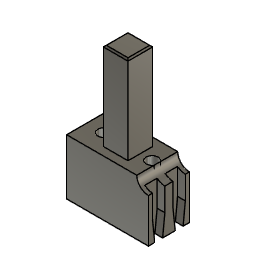
Wheel truing stand (copy) (Autodesk Fusion 360 archive; units mm, degrees)
design "Non_movable_piece"
Autodesk Fusion 360 part; units mm, degrees
(part 1 of 2)
sketch "Sketch1" plane through (0, 0, 0) normal (0, 1, 0) x (1, 0, 0)
  line L0 (0, 0) -> (56, 0)
  line L1 (56, 0) -> (56, -38)
  line L2 (56, -38) -> (0, -38)
  line L3 (0, -38) -> (0, 0)
  line L4 (56, 0) -> (56, -1.6379)
  line L5 (56, 0) -> (56, -30)
  circle A0 centre (56, -38) radius 8
  dimension "d1" = 56
  dimension "d2" = 38
  dimension "d5" = 30
  constraint horizontal L0
  constraint vertical L1
  constraint horizontal L2
  constraint vertical L3
  constraint coincident L0.start L3.end
  constraint coincident L1 L4.end
  constraint perpendicular L0 L5
  constraint coincident L1.end L2.start
  constraint coincident L5.end A0
  measures "d1" distance of L0.start L0.end
  measures "d2" distance of L0.start L2.end
  measures "d5" distance of L0.end L5.end
  measures "d8" distance of L0.start
  measures "d9" distance of L0.start
extrude "Extrude1" add sketch "Sketch1" along normal blind 28 contours L0 L1 L2 L3 L4 L5 A0
sketch "Sketch3" plane through (0, 0, 38) normal (0, 0, 1) x (-1, 0, 0)
  line L0 (0, 0) -> (-48, 0)
  line L1 (-48, 0) -> (-48, -28)
  line L2 (-48, -28) -> (0, -28)
  line L3 (0, -28) -> (0, 0)
  line L4 (0, -28) -> (-56, -28)
  line L5 (-56, -28) -> (-56, 0)
  line L6 (-56, 0) -> (0, 0)
  line L7 (0, 0) -> (0, -28)
  line L8 (-56, -28) -> (0, 0) construction
  line L9 (0, -28) -> (-56, 0) construction
  line L10 (-36.4, -5.6) -> (-19.6, -5.6)
  line L11 (-19.6, -5.6) -> (-19.6, -22.4)
  line L12 (-19.6, -22.4) -> (-36.4, -22.4)
  line L13 (-36.4, -22.4) -> (-36.4, -5.6)
  line L14 (-36.4, -5.6) -> (-19.6, -22.4) construction
  line L15 (-19.6, -5.6) -> (-36.4, -22.4) construction
  line L16 (0, -14) -> (-56, -14) construction
  line L17 (0, -14) -> (-11.5, -14)
  line L18 (-56, -14) -> (-44.5, -14)
  circle A0 centre (-11.5, -14) radius 2
  line L19 (-28, 0) -> (-28, -28) construction
  circle A1 centre (-44.5, -14) radius 2
  circle A2 centre (-11.5, -14) radius 4.1
  circle A3 centre (-44.5, -14) radius 4.1
  line L20 (-38.15, -3.85) -> (-17.85, -3.85)
  line L21 (-17.85, -3.85) -> (-17.85, -24.15)
  line L22 (-17.85, -24.15) -> (-38.15, -24.15)
  line L23 (-38.15, -24.15) -> (-38.15, -3.85)
  line L24 (-38.15, -3.85) -> (-17.85, -24.15) construction
  line L25 (-17.85, -3.85) -> (-38.15, -24.15) construction
  line L26 (-16.35, -2.35) -> (-16.35, -25.65)
  line L27 (-16.35, -25.65) -> (-39.65, -25.65)
  line L28 (-39.65, -25.65) -> (-39.65, -2.35)
  line L29 (-39.65, -2.35) -> (-16.35, -2.35)
  point P0 (-28, -14)
  point P1 (-28, -14)
  dimension "d6" = 56
  dimension "d7" = 28
  dimension "d8" = 16.8
  dimension "d9" = 16.8
  dimension "d13" = 11.5
  dimension "d14" = 11.5
  dimension "d15" = 4
  dimension "d17" = 8.2
  dimension "d33" = 20.3
  dimension "d34" = 20.3
  dimension "d35" = -1.5
  constraint horizontal L4
  constraint vertical L5
  constraint horizontal L6
  constraint vertical L7
  constraint coincident L2.end L3.start
  constraint coincident L0.start L3.end
  constraint horizontal L10
  constraint perpendicular L10 L11
  constraint parallel L10 L12
  constraint parallel L11 L13
  constraint coincident L14 P1
  constraint coincident L15 P1
  constraint midpoint L8 P1
  constraint midpoint L7 L16.start
  constraint midpoint L5 L16.end
  constraint perpendicular L11 L17
  constraint perpendicular L1 L18
  constraint coincident L17.end A0.centre
  constraint midpoint L6 L19.start
  constraint midpoint L4 L19.end
  constraint symmetric A0 L19 A1
  constraint symmetric L19 A2 A3
  constraint horizontal L20
  constraint perpendicular L20 L21
  constraint parallel L20 L22
  constraint parallel L21 L23
  constraint coincident L24 P1
  constraint coincident L25 P1
  constraint coincident P1 P0
  measures "d6" distance of L5 L7
  measures "d7" distance of L4 L6
  measures "d8" distance of L11.end L12.end
  measures "d9" distance of L10.end L11.end
  measures "d13" distance of L16.start L17.end
  measures "d14" distance of L16.end L18.end
  measures "d15" diameter of A0
  measures "d17" diameter of A2
  measures "d33" distance of L21.end L22.end
  measures "d34" distance of L20.end L21.end
extrude "Extrude3" cut sketch "Sketch3" against normal blind 38 contours A0 | A1
extrude "Extrude2" add sketch "Sketch3" along normal blind 60 contours L10 L11 L12 L13
chamfer "Chamfer1" distance 1 angle 45 4 edges at (28, 5.6, 98) (19.6, 14, 98) (28, 22.4, 98) (36.4, 14, 98)
extrude "Extrude4" cut sketch "Sketch3" against normal blind 32 contours L1 A3 | A2
chamfer "Chamfer2" distance 1.8 angle 45 2 edges at (13.3647, 14.7232, 6) (46.3647, 14.7232, 6)
sketch "Sketch4" plane through (56, 0, 0) normal (1, 0, 0) x (0, 1, 0)
  line L0 (0, 30) -> (0, 0)
  line L1 (0, 0) -> (28, 0)
  line L2 (28, 0) -> (28, 30)
  line L3 (28, 30) -> (0, 30)
  line L4 (0, 38) -> (28, 38) construction
  line L5 (28, 38) -> (28, 0) construction
  line L6 (28, 0) -> (0, 0) construction
  line L7 (0, 0) -> (0, 38) construction
  line L8 (14, 0) -> (14, 38) construction
  line L9 (7, 0) -> (7, 38) construction
  line L10 (7, 0) -> (4.5, 0)
  line L11 (7, 14) -> (3, 14)
  line L12 (3, 14) -> (4.5, 0)
  line L13 (7, 14) -> (11, 14)
  line L14 (11, 14) -> (9.5, 0)
  line L15 (7, 0) -> (9.5, 0)
  line L16 (7, 14.2) -> (2.7774, 14.2)
  line L17 (2.7774, 14.2) -> (4.3203, -0.2)
  line L18 (7, -0.2) -> (4.3203, -0.2)
  line L19 (7, -0.2) -> (9.6797, -0.2)
  line L20 (11.2226, 14.2) -> (9.6797, -0.2)
  line L21 (7, 14.2) -> (11.2226, 14.2)
  line L22 (2.7774, 14.2) -> (2.7774, 38)
  line L23 (11.2226, 14.2) -> (11.2226, 38.0127)
  line L24 (16.7774, 14.2) -> (16.7774, 38.0127)
  line L25 (25.2226, 14.2) -> (25.2226, 38)
  line L26 (16.7774, 14.2) -> (18.3203, -0.2)
  line L27 (25.2226, 14.2) -> (23.6797, -0.2)
  line L28 (21, -0.2) -> (23.6797, -0.2)
  line L29 (21, -0.2) -> (18.3203, -0.2)
  line L30 (16.7774, 38.0127) -> (25.2226, 38)
  line L31 (11.2226, 38.0127) -> (2.7774, 38)
  dimension "d24" = 2.5
  dimension "d25" = 4
  dimension "d27" = 14
  dimension "d28" = 0.2
  dimension "d29" = 180
  dimension "d30" = 23.8127
  constraint horizontal L4
  constraint vertical L5
  constraint horizontal L6
  constraint vertical L7
  constraint coincident L1.end L2.start
  constraint midpoint L1 L8.start
  constraint midpoint L4 L8.end
  constraint perpendicular L4 L8
  constraint coincident L1 L9.start
  constraint coincident L4 L9.end
  constraint perpendicular L4 L9
  constraint perpendicular L9 L10
  constraint coincident L9 L11.start
  constraint perpendicular L9 L11
  constraint symmetric L10.start L9 L15.start
  constraint symmetric L9 L10.end L14.end
  constraint symmetric L9 L11.start L13.start
  constraint symmetric L9 L11.end L13.end
  constraint vertical L22
  constraint coincident L4 L22.end
  constraint symmetric L8 L16.end L25.start
  constraint symmetric L8 L17.end L27.end
  constraint symmetric L8 L18.start L28.start
  constraint symmetric L8 L19.end L26.end
  constraint symmetric L8 L20.start L24.start
  constraint symmetric L8 L22.end L25.end
  constraint symmetric L8 L23.end L24.end
  measures "d24" distance of L9.start L10.end
  measures "d25" distance of L11.start L11.end
  measures "d27" distance of L10 L11
  measures "d29" angle of L22 L23
  measures "d30" distance of L20.start L23.end
extrude "Extrude5" cut sketch "Sketch4" against normal blind 5.3 contours L3 L22 L23 L31 | L3 L16 L21 L22 L23 | L1 L11 L12 L13 L14 L16 L17 L20 L21 | L1 L10 L11 L12 L13 L14 L15 | L3 L24 L25 L30 | L1 L3 L24 L25 L26 L27
equation "d13 = ( 23 / 2 ) * 1 mm"
equation "d14 = ( 23 / 2 ) * 1 mm"

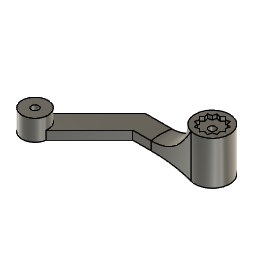
design "wheel_aligment_arm_right_20mm_offset"
Autodesk Fusion 360 part; units mm, degrees
sketch "Sketch1" plane through (0, 0, 0) normal (0, 0, 1) x (1, 0, 0)
  line L0 (0, 0) -> (40, 0)
  line L1 (40, 12) -> (0, 12)
  line L2 (0, 12) -> (0, 0)
  line L3 (40, 0) -> (68.2843, -28.2843)
  line L4 (40, 0) -> (80, 0) construction
  line L5 (68.2843, -28.2843) -> (76.7696, -19.799)
  line L6 (76.7696, -19.799) -> (44.9706, 12)
  line L7 (40, 12) -> (44.9706, 12)
  circle A0 centre (0, 6) radius 10
  line L8 (0, 6) -> (0, 13.5) construction
  line L9 (0, 13.5) -> (0, -1.5) construction
  line L10 (0, 6) -> (7.5, 6) construction
  line L11 (7.5, 6) -> (-7.5, 6) construction
  line L12 (-7.5, 6) -> (0, 13.5)
  line L13 (0, 13.5) -> (7.5, 6)
  line L14 (7.5, 6) -> (0, -1.5)
  line L15 (0, -1.5) -> (-7.5, 6)
  line L16 (0, 6) -> (3.75, 12.4952) construction
  line L17 (3.75, 12.4952) -> (-3.75, -0.4952) construction
  line L18 (0, 6) -> (6.4952, 2.25) construction
  line L19 (6.4952, 2.25) -> (-6.4952, 9.75) construction
  line L20 (-6.4952, 9.75) -> (3.75, 12.4952)
  line L21 (3.75, 12.4952) -> (6.4952, 2.25)
  line L22 (6.4952, 2.25) -> (-3.75, -0.4952)
  line L23 (-3.75, -0.4952) -> (-6.4952, 9.75)
  line L24 (0, 6) -> (6.4952, 9.75) construction
  line L25 (0, 6) -> (7.5, 6) construction
  line L26 (6.4952, 9.75) -> (-6.4952, 2.25) construction
  line L27 (0, 6) -> (3.75, -0.4952) construction
  line L28 (3.75, -0.4952) -> (-3.75, 12.4952) construction
  line L29 (-3.75, 12.4952) -> (-6.4952, 2.25)
  line L30 (-6.4952, 2.25) -> (3.75, -0.4952)
  line L31 (3.75, -0.4952) -> (6.4952, 9.75)
  line L32 (6.4952, 9.75) -> (-3.75, 12.4952)
  circle A1 centre (0, 6) radius 2
  circle A2 centre (72.5269, -24.0416) radius 7.5
  line L33 (76.1769, -26.149) -> (76.1769, -21.9343)
  line L34 (76.1769, -21.9343) -> (72.5269, -19.827)
  line L35 (72.5269, -19.827) -> (68.8769, -21.9343)
  line L36 (68.8769, -21.9343) -> (68.8769, -26.149)
  line L37 (68.8769, -26.149) -> (72.5269, -28.2563)
  line L38 (72.5269, -28.2563) -> (76.1769, -26.149)
  line L39 (68.8769, -21.9343) -> (68.8769, -17.4897)
  line L40 (76.1769, -21.9343) -> (76.1769, -17.4897)
  circle A3 centre (72.5269, -24.0416) radius 2.1
  point P0 (72.5269, -24.0416)
  dimension "d1" = 40
  dimension "d2" = 12
  dimension "d3" = 40
  dimension "d4" = 45
  dimension "d5" = 12
  dimension "d8" = 7.5
  dimension "d9" = 15
  dimension "d10" = 7.5
  dimension "d11" = 15
  dimension "d12" = 7.5
  dimension "d13" = 30
  dimension "d14" = 15
  dimension "d15" = 7.5
  dimension "d16" = 90
  dimension "d17" = 15
  dimension "d18" = 30
  dimension "d19" = 7.5
  dimension "d20" = 15
  dimension "d21" = 7.5
  dimension "d22" = 15
  dimension "d23" = 20
  dimension "d24" = 4
  dimension "d25" = 15
  dimension "d35" = 3.65
  dimension "d39" = 4.2
  dimension "d42" = 180
  constraint horizontal L0
  constraint horizontal L1
  constraint vertical L2
  constraint coincident L0.start L2.end
  constraint horizontal L4
  constraint perpendicular L3 L5
  constraint perpendicular L5 L6
  constraint midpoint L2 A0.centre
  constraint coincident A0.centre L8.start
  constraint parallel L2 L8
  constraint perpendicular L0 L9
  constraint perpendicular L8 L10
  constraint parallel L10 L11
  constraint parallel L16 L17
  constraint perpendicular L16 L19
  constraint horizontal L25
  constraint parallel L24 L26
  constraint perpendicular L24 L27
  constraint parallel L27 L28
  constraint midpoint L5 P0
  constraint coincident P0 A2.centre
  constraint vertical L39
  constraint coincident A2 L39.end
  constraint vertical L40
  constraint coincident A2 L40.end
  measures "d1" distance of L0.start L0.end
  measures "d2" distance of L0.start L1.end
  measures "d3" distance of L0.end L3.end
  measures "d4" angle of L3 L4
  measures "d5" distance of L3.end L5.end
  measures "d8" distance of A0.centre L8.end
  measures "d9" distance of L8.end L9.end
  measures "d10" distance of A0.centre L10.end
  measures "d11" distance of L10.end L11.end
  measures "d12" distance of A0.centre L16.end
  measures "d13" angle of L9 L16
  measures "d14" distance of L16.end L17.end
  measures "d15" distance of A0.centre L18.end
  measures "d16" angle of L17 L18
  measures "d17" distance of L18.end L19.end
  measures "d18" angle of L24 L25
  measures "d19" distance of A0.centre L24.end
  measures "d20" distance of L24.end L26.end
  measures "d21" distance of A0.centre L27.end
  measures "d22" distance of L27.end L28.end
  measures "d23" diameter of A0
  measures "d24" diameter of A1
  measures "d25" diameter of A2
  measures "d35" distance of P0 L38
  measures "d39" diameter of A3
  measures "d42" angle of L36 L39 L0.start
extrude "Extrude1" add sketch "Sketch1" against normal blind 5
extrude "Extrude9" add sketch "Sketch1" against normal blind 25 contours L0 L2 L14 L30 | L0 L2 L14 L15 L22 | L0 L14 L30 | L0 L1 A0 L12 L13 L14 L15 L20 L21 L22 L23 L29 L30 L31 L32 | L2 L12 L15 L20 L23 L29 L30 A1 | L2 L13 L14 L21 L22 L31 L32 A1 | L15 L22 L30 | L14 L22 L30 | L0 L14 L22 L30 L31 | L0 L30 L31 | L2 A1 | L2 A1 | L14 L22 L31 | L15 L22 L23 L30 | L15 L23 L30 | L0 L1 A0 L13 L14 L21 L22 L31 L32 | L14 L21 L31 | L14 L21 L22 L31 | L15 L23 L29 L30 | L15 L23 L29 | L1 L2 L12 L13 L32 | L1 L2 L13 L20 | L13 L20 L32 | L12 L20 L32 | L13 L14 L21 L31 | L13 L21 L31 | L12 L15 L23 L29 | L12 L23 L29 | L12 L20 L29 L32 | L12 L20 L29 | L1 L13 L20 L21 L32 | L1 L13 L20 | L13 L21 L32 | L13 L21 L31 L32 | L12 L20 L23 L29 | L1 L20 L21
extrude "Extrude2" cut sketch "Sketch1" along normal blind 2.2 from surface at -25 contours L0 L2 L14 L30 | L0 L2 L14 L15 L22 | L0 L14 L30 | L2 L12 L15 L20 L23 L29 L30 A1 | L2 L13 L14 L21 L22 L31 L32 A1 | L15 L22 L30 | L14 L22 L30 | L0 L14 L22 L30 L31 | L0 L30 L31 | L2 A1 | L2 A1 | L14 L22 L31 | L15 L22 L23 L30 | L15 L23 L30 | L14 L21 L31 | L14 L21 L22 L31 | L15 L23 L29 L30 | L15 L23 L29 | L1 L2 L12 L13 L32 | L1 L2 L13 L20 | L13 L20 L32 | L12 L20 L32 | L13 L14 L21 L31 | L13 L21 L31 | L12 L15 L23 L29 | L12 L23 L29 | L12 L20 L29 L32 | L12 L20 L29 | L1 L13 L20 L21 L32 | L1 L13 L20 | L13 L21 L32 | L13 L21 L31 L32 | L12 L20 L23 L29 | L1 L20 L21
extrude "Extrude3" cut sketch "Sketch1" against normal blind 25 contours L2 A1 | L2 A1
extrude "Extrude4" add sketch "Sketch1" against normal blind 12 contours L3 L5 A2 L36 L37 L39 | L3 L5 L6 A2 L33 L37 L38 L40 | L5 L6 A2 L34 L35 L39 L40 | L5 L34 L35 L36 L37 A3 | L5 L33 L34 L37 L38 A3 | L6 A2 L40 | L5 A3 | L5 A3 | L5 L6 L40 | L5 L34 L40
extrude "Extrude5" cut sketch "Sketch1" along normal mid plane 4 from surface at -7 contours L5 L6 A2 L34 L35 L39 L40 | L5 L34 L35 L36 L37 A3 | L5 L33 L34 L37 L38 A3 | L6 A2 L40 | L5 A3 | L5 A3 | L5 L34 L40
extrude "Extrude6" cut sketch "Sketch1" against normal blind 12 contours L5 A3 | L5 A3
move_body "Move1" bodies 1 to x (-1, 0, 0) y (0, 1, 0) z (0, 0, -1) at (-20, 0, -50)
move_body "Move2" bodies 1 to x (1, 0, 0) y (0, 1, 0) z (0, 0, 1) at (20, 0, 50)
move_body "Move3" bodies 1 to x (1, 0, 0) y (0, 1, 0) z (0, 0, 1) at (-0.21, 0.1034, 0.1851)
fillet "Fillet1" radius 20 1 edges at (-10.21, 6.1034, 5.1851)
fillet "Fillet2" radius 100 2 edges at (-8.21, 0.1034, 12.6851) (-8.21, 12.1034, 12.6851)
equation "d13 = ( 90 / 3 ) * 1 deg"

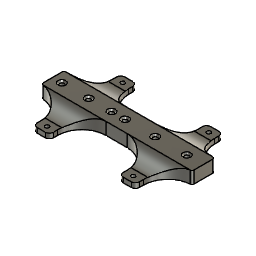
design "base"
Autodesk Fusion 360 part; units mm, degrees
sketch "Sketch1" plane through (0, 0, 0) normal (0, 0, 1) x (1, 0, 0)
  line L0 (0, 0) -> (186, 0)
  line L1 (186, 0) -> (186, 28)
  line L2 (186, 28) -> (0, 28)
  line L3 (0, 28) -> (0, 0)
  line L4 (0, 14) -> (186, 14) construction
  circle A0 centre (11.5, 14) radius 2.75
  circle A1 centre (44.5, 14) radius 2.75
  circle A2 centre (72.6667, 14) radius 2.75
  circle A3 centre (89.3333, 14) radius 2.75
  circle A4 centre (126.5, 14) radius 2.75
  circle A5 centre (165.5, 14) radius 2.75
  line L5 (13.8094, 10) -> (16.1188, 14)
  line L6 (16.1188, 14) -> (13.8094, 18)
  line L7 (13.8094, 18) -> (9.1906, 18)
  line L8 (9.1906, 18) -> (6.8812, 14)
  line L9 (6.8812, 14) -> (9.1906, 10)
  line L10 (9.1906, 10) -> (13.8094, 10)
  line L11 (46.8094, 10) -> (49.1188, 14)
  line L12 (49.1188, 14) -> (46.8094, 18)
  line L13 (46.8094, 18) -> (42.1906, 18)
  line L14 (42.1906, 18) -> (39.8812, 14)
  line L15 (39.8812, 14) -> (42.1906, 10)
  line L16 (42.1906, 10) -> (46.8094, 10)
  line L17 (74.9761, 10) -> (77.2855, 14)
  line L18 (77.2855, 14) -> (74.9761, 18)
  line L19 (74.9761, 18) -> (70.3573, 18)
  line L20 (70.3573, 18) -> (68.0479, 14)
  line L21 (68.0479, 14) -> (70.3573, 10)
  line L22 (70.3573, 10) -> (74.9761, 10)
  line L23 (91.6427, 10) -> (93.9521, 14)
  line L24 (93.9521, 14) -> (91.6427, 18)
  line L25 (91.6427, 18) -> (87.0239, 18)
  line L26 (87.0239, 18) -> (84.7145, 14)
  line L27 (84.7145, 14) -> (87.0239, 10)
  line L28 (87.0239, 10) -> (91.6427, 10)
  line L29 (128.8094, 10) -> (131.1188, 14)
  line L30 (131.1188, 14) -> (128.8094, 18)
  line L31 (128.8094, 18) -> (124.1906, 18)
  line L32 (124.1906, 18) -> (121.8812, 14)
  line L33 (121.8812, 14) -> (124.1906, 10)
  line L34 (124.1906, 10) -> (128.8094, 10)
  line L35 (167.8094, 10) -> (170.1188, 14)
  line L36 (170.1188, 14) -> (167.8094, 18)
  line L37 (167.8094, 18) -> (163.1906, 18)
  line L38 (163.1906, 18) -> (160.8812, 14)
  line L39 (160.8812, 14) -> (163.1906, 10)
  line L40 (163.1906, 10) -> (167.8094, 10)
  point P0 (11.5, 14)
  point P1 (44.5, 14)
  point P2 (72.6667, 14)
  point P3 (89.3333, 14)
  point P4 (126.5, 14)
  point P5 (165.5, 14)
  dimension "d1" = 186
  dimension "d2" = 28
  dimension "d3" = 5.5
  dimension "d4" = 11.5
  dimension "d5" = 5.5
  dimension "d6" = 44.5
  dimension "d7" = 5.5
  dimension "d8" = 5.5
  dimension "d9" = 5.5
  dimension "d10" = 5.5
  dimension "d11" = 72.6667
  dimension "d12" = 89.3333
  dimension "d13" = 20.5
  dimension "d14" = 126.5
  dimension "d18" = 4
  dimension "d19" = 4
  dimension "d20" = 4
  dimension "d21" = 4
  dimension "d22" = 4
  dimension "d23" = 4
  constraint horizontal L0
  constraint vertical L1
  constraint horizontal L2
  constraint vertical L3
  constraint coincident L0.start L3.end
  constraint midpoint L3 L4.start
  constraint midpoint L1 L4.end
  constraint coincident L4 P0
  constraint coincident L4 P1
  constraint coincident L4 P2
  constraint coincident L4 P3
  constraint coincident L4 P4
  constraint coincident L4 P5
  constraint coincident P0 A0.centre
  constraint coincident P1 A1.centre
  constraint coincident P2 A2.centre
  constraint coincident P3 A3.centre
  constraint coincident P4 A4.centre
  constraint coincident P5 A5.centre
  measures "d1" distance of L0.start L0.end
  measures "d2" distance of L0.start L2.end
  measures "d3" diameter of A0
  measures "d4" distance of L4.start P0
  measures "d5" diameter of A1
  measures "d6" distance of L3 P1
  measures "d7" diameter of A2
  measures "d8" diameter of A3
  measures "d9" diameter of A4
  measures "d10" diameter of A5
  measures "d11" distance of L3 P2
  measures "d12" distance of L3 P3 L0.start
  measures "d13" distance of L1 P5
  measures "d14" distance of L3 P4
  measures "d18" distance of P0 L10
  measures "d19" distance of P1 L16
  measures "d20" distance of P2 L22
  measures "d21" distance of P3 L28
  measures "d22" distance of P4 L34
  measures "d23" distance of P5 L40
extrude "Extrude1" add sketch "Sketch1" along normal blind 15 contours L0 L1 L2 L3 | L5 L6 L7 L8 L9 L10 | L11 L12 L13 L14 L15 L16 | L17 L18 L19 L20 L21 L22 | L23 L24 L25 L26 L27 L28 | L29 L30 L31 L32 L33 L34 | L35 L36 L37 L38 L39 L40
chamfer "Chamfer1" distance 2 angle 45 6 edges at (8.9361, 14.9944, 15) (41.9361, 14.9944, 15) (70.1028, 14.9944, 15) (86.7694, 14.9944, 15) (123.9361, 14.9944, 15) (162.9361, 14.9944, 15)
extrude "Extrude2" cut sketch "Sketch1" along normal blind 4 contours L5 L6 L7 L8 L9 L10 | L11 L12 L13 L14 L15 L16 | L17 L18 L19 L20 L21 L22 | L23 L24 L25 L26 L27 L28 | L29 L30 L31 L32 L33 L34 | L35 L36 L37 L38 L39 L40
sketch "Sketch2" plane through (0, 0, 0) normal (-1, 0, 0) x (0, -1, 0)
  line L0 (-28, 0) -> (0, 0)
  line L1 (0, 0) -> (0, 15)
  line L2 (0, 15) -> (-28, 15)
  line L3 (-28, 15) -> (-28, 0)
  line L4 (0, 0) -> (40, 0)
  line L5 (40, 0) -> (40, 6)
  line L6 (40, 6) -> (25, 6)
  arc A0 (0, 15) -> (25, 6) centre (25, 45.2222) ccw
  line L7 (0, 15) -> (-28, 0) construction
  line L8 (-28, 15) -> (0, 0) construction
  line L9 (-14, -17.2562) -> (-14, 34) construction
  line L10 (-28, 0) -> (-68, 0)
  arc A1 (-53, 6) -> (-28, 15) centre (-53, 45.2222) ccw
  line L11 (-68, 6) -> (-53, 6)
  line L12 (-68, 0) -> (-68, 6)
  dimension "d26" = 40
  constraint coincident L0.end L1.start
  constraint perpendicular L1 L4
  constraint perpendicular L4 L5
  constraint perpendicular L5 L6
  constraint tangent L6 A0
  constraint coincident L1.end L2.start
  constraint coincident L0.start L3.end
  constraint coincident L2.end L3.start
  constraint perpendicular L2 L9
  constraint symmetric L0.end L9 L0.start
  constraint symmetric L4.end L9 L10.end
  constraint symmetric L5.end L9 L11.start
  constraint symmetric L6.end L9 A1.start
  constraint symmetric L1.end L9 L2.end
  constraint symmetric A0 L9 A1
  measures "d26" distance of L0.end L4.end
extrude "Extrude3" add sketch "Sketch2" against normal blind 20 from surface at -30 contours L3 L10 A1 L11 L12 | L1 L4 L5 L6 A0
extrude "Extrude4" add sketch "Sketch2" along normal blind 20 from surface at -156 contours L3 L10 A1 L11 L12 | L1 L4 L5 L6 A0
fillet "Fillet1" radius 30 8 edges at (50, 0, 7.5) (30, 0, 7.5) (50, 28, 7.5) (136, 28, 7.5) (156, 28, 7.5) (156, 0, 7.5) (136, 0, 7.5) (30, 28, 7.5)
sketch "Sketch3" plane through (0, 0, 6) normal (0, 0, 1) x (-1, 0, 0)
  line L0 (-30, 30) -> (-30, 40)
  line L1 (-30, 40) -> (-50, 40)
  line L2 (-50, 40) -> (-50, 30)
  arc A0 (-50.4196, 25) -> (-50, 30) centre (-80, 30) ccw
  line L3 (-50.4196, 25) -> (-29.5804, 25)
  arc A1 (-30, 30) -> (-29.5804, 25) centre (0, 30) ccw
  line L4 (-156, 40) -> (-156, 30)
  arc A2 (-156.4196, 25) -> (-156, 30) centre (-186, 30) ccw
  line L5 (-156.4196, 25) -> (-135.5804, 25)
  arc A3 (-136, 30) -> (-135.5804, 25) centre (-106, 30) ccw
  line L6 (-136, 30) -> (-136, 40)
  line L7 (-136, 40) -> (-156, 40)
  line L8 (-156, -58) -> (-156, -68)
  line L9 (-156, -68) -> (-136, -68)
  line L10 (-136, -68) -> (-136, -58)
  arc A4 (-135.5804, -53) -> (-136, -58) centre (-106, -58) ccw
  line L11 (-135.5804, -53) -> (-156.4196, -53)
  arc A5 (-156, -58) -> (-156.4196, -53) centre (-186, -58) ccw
  line L12 (-30, -68) -> (-30, -58)
  arc A6 (-29.5804, -53) -> (-30, -58) centre (0, -58) ccw
  line L13 (-29.5804, -53) -> (-50.4196, -53)
  arc A7 (-50, -58) -> (-50.4196, -53) centre (-80, -58) ccw
  line L14 (-50, -58) -> (-50, -68)
  line L15 (-50, -68) -> (-30, -68)
  line L16 (-50.4196, 25) -> (-30, 40) construction
  line L17 (-29.5804, 25) -> (-50, 40) construction
  line L18 (-156, -68) -> (-135.5804, -53) construction
  line L19 (-136, -68) -> (-156.4196, -53) construction
  line L20 (-136, 40) -> (-156.4196, 25) construction
  line L21 (-135.5804, 25) -> (-156, 40) construction
  line L22 (-29.5804, -53) -> (-50, -68) construction
  line L23 (-30, -68) -> (-50.4196, -53) construction
  circle A8 centre (-40, -60.6541) radius 2.5
  circle A9 centre (-40, 32.6541) radius 2.5
  circle A10 centre (-146, 32.6541) radius 2.5
  circle A11 centre (-146, -60.6541) radius 2.5
  point P0 (-146, 32.6541)
  point P1 (-146, -60.6541)
  dimension "d35" = 5
  dimension "d36" = 5
  dimension "d37" = 5
  dimension "d38" = 5
  constraint coincident A0.start L3.start
  constraint coincident L0.end L1.start
  constraint coincident L3.end A1.end
  constraint coincident L1.end L2.start
  constraint coincident L8.end L9.start
  constraint coincident A4.start L11.start
  constraint coincident L9.end L10.start
  constraint coincident L11.end A5.end
  constraint coincident L6.end L7.start
  constraint coincident A2.start L5.start
  constraint coincident L5.end A3.end
  constraint coincident L4.start L7.end
  constraint coincident L21 P0
  constraint coincident L20 P0
  constraint coincident L18 P1
  constraint coincident L19 P1
  constraint coincident A6.start L13.start
  constraint coincident L14.end L15.start
  constraint coincident L12.start L15.end
  constraint coincident L13.end A7.end
  constraint coincident L22 A8.centre
  constraint coincident L23 A8.centre
  constraint coincident L17 A9.centre
  constraint coincident L16 A9.centre
  constraint coincident P0 A10.centre
  constraint coincident P1 A11.centre
  measures "d35" diameter of A8
  measures "d36" diameter of A9
  measures "d37" diameter of A10
  measures "d38" diameter of A11
extrude "Extrude5" cut sketch "Sketch3" against normal blind 6 contours A8 | A9 | A10 | A11
fillet "Fillet2" radius 2.5 4 edges at (186, 0, 7.5) (186, 28, 7.5) (0, 0, 7.5) (0, 28, 7.5)
fillet "Fillet3" radius 5 8 edges at (30, -40, 3) (50, -40, 3) (136, -40, 3) (156, -40, 3) (156, 68, 3) (136, 68, 3) (50, 68, 3) (30, 68, 3)
equation "d1 = 50 mm + 56 mm + 80 mm"
equation "d11 = 56 mm + ( 50 / 3 ) * 1 mm"
equation "d12 = 56 mm + ( 2 * 50 / 3 ) * 1 mm"
equation "d14 = 106 mm + 20.5 mm"
equation "d30 = -186 mm + 30.00 mm"

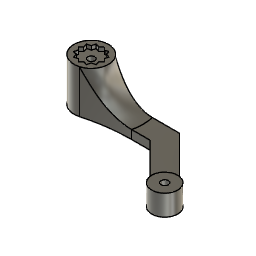
design "wheel_aligment_arm_left_20mm_offset"
Autodesk Fusion 360 part; units mm, degrees
sketch "Sketch1" plane through (0, 0, 0) normal (0, 0, 1) x (1, 0, 0)
  line L0 (0, 0) -> (40, 0)
  line L1 (40, 12) -> (0, 12)
  line L2 (0, 12) -> (0, 0)
  line L3 (40, 0) -> (68.2843, -28.2843)
  line L4 (40, 0) -> (80, 0) construction
  line L5 (68.2843, -28.2843) -> (76.7696, -19.799)
  line L6 (76.7696, -19.799) -> (44.9706, 12)
  line L7 (40, 12) -> (44.9706, 12)
  circle A0 centre (0, 6) radius 10
  line L8 (0, 6) -> (0, 13.5) construction
  line L9 (0, 13.5) -> (0, -1.5) construction
  line L10 (0, 6) -> (7.5, 6) construction
  line L11 (7.5, 6) -> (-7.5, 6) construction
  line L12 (-7.5, 6) -> (0, 13.5)
  line L13 (0, 13.5) -> (7.5, 6)
  line L14 (7.5, 6) -> (0, -1.5)
  line L15 (0, -1.5) -> (-7.5, 6)
  line L16 (0, 6) -> (3.75, 12.4952) construction
  line L17 (3.75, 12.4952) -> (-3.75, -0.4952) construction
  line L18 (0, 6) -> (6.4952, 2.25) construction
  line L19 (6.4952, 2.25) -> (-6.4952, 9.75) construction
  line L20 (-6.4952, 9.75) -> (3.75, 12.4952)
  line L21 (3.75, 12.4952) -> (6.4952, 2.25)
  line L22 (6.4952, 2.25) -> (-3.75, -0.4952)
  line L23 (-3.75, -0.4952) -> (-6.4952, 9.75)
  line L24 (0, 6) -> (6.4952, 9.75) construction
  line L25 (0, 6) -> (7.5, 6) construction
  line L26 (6.4952, 9.75) -> (-6.4952, 2.25) construction
  line L27 (0, 6) -> (3.75, -0.4952) construction
  line L28 (3.75, -0.4952) -> (-3.75, 12.4952) construction
  line L29 (-3.75, 12.4952) -> (-6.4952, 2.25)
  line L30 (-6.4952, 2.25) -> (3.75, -0.4952)
  line L31 (3.75, -0.4952) -> (6.4952, 9.75)
  line L32 (6.4952, 9.75) -> (-3.75, 12.4952)
  circle A1 centre (0, 6) radius 2
  circle A2 centre (72.5269, -24.0416) radius 7.5
  line L33 (76.1769, -26.149) -> (76.1769, -21.9343)
  line L34 (76.1769, -21.9343) -> (72.5269, -19.827)
  line L35 (72.5269, -19.827) -> (68.8769, -21.9343)
  line L36 (68.8769, -21.9343) -> (68.8769, -26.149)
  line L37 (68.8769, -26.149) -> (72.5269, -28.2563)
  line L38 (72.5269, -28.2563) -> (76.1769, -26.149)
  line L39 (68.8769, -21.9343) -> (68.8769, -17.4897)
  line L40 (76.1769, -21.9343) -> (76.1769, -17.4897)
  circle A3 centre (72.5269, -24.0416) radius 2.1
  point P0 (72.5269, -24.0416)
  dimension "d1" = 40
  dimension "d2" = 12
  dimension "d3" = 40
  dimension "d4" = 45
  dimension "d5" = 12
  dimension "d8" = 7.5
  dimension "d9" = 15
  dimension "d10" = 7.5
  dimension "d11" = 15
  dimension "d12" = 7.5
  dimension "d13" = 30
  dimension "d14" = 15
  dimension "d15" = 7.5
  dimension "d16" = 90
  dimension "d17" = 15
  dimension "d18" = 30
  dimension "d19" = 7.5
  dimension "d20" = 15
  dimension "d21" = 7.5
  dimension "d22" = 15
  dimension "d23" = 20
  dimension "d24" = 4
  dimension "d25" = 15
  dimension "d35" = 3.65
  dimension "d39" = 4.2
  dimension "d42" = 180
  constraint horizontal L0
  constraint horizontal L1
  constraint vertical L2
  constraint coincident L0.start L2.end
  constraint horizontal L4
  constraint perpendicular L3 L5
  constraint perpendicular L5 L6
  constraint midpoint L2 A0.centre
  constraint coincident A0.centre L8.start
  constraint parallel L2 L8
  constraint perpendicular L0 L9
  constraint perpendicular L8 L10
  constraint parallel L10 L11
  constraint parallel L16 L17
  constraint perpendicular L16 L19
  constraint horizontal L25
  constraint parallel L24 L26
  constraint perpendicular L24 L27
  constraint parallel L27 L28
  constraint midpoint L5 P0
  constraint coincident P0 A2.centre
  constraint vertical L39
  constraint coincident A2 L39.end
  constraint vertical L40
  constraint coincident A2 L40.end
  measures "d1" distance of L0.start L0.end
  measures "d2" distance of L0.start L1.end
  measures "d3" distance of L0.end L3.end
  measures "d4" angle of L3 L4
  measures "d5" distance of L3.end L5.end
  measures "d8" distance of A0.centre L8.end
  measures "d9" distance of L8.end L9.end
  measures "d10" distance of A0.centre L10.end
  measures "d11" distance of L10.end L11.end
  measures "d12" distance of A0.centre L16.end
  measures "d13" angle of L9 L16
  measures "d14" distance of L16.end L17.end
  measures "d15" distance of A0.centre L18.end
  measures "d16" angle of L17 L18
  measures "d17" distance of L18.end L19.end
  measures "d18" angle of L24 L25
  measures "d19" distance of A0.centre L24.end
  measures "d20" distance of L24.end L26.end
  measures "d21" distance of A0.centre L27.end
  measures "d22" distance of L27.end L28.end
  measures "d23" diameter of A0
  measures "d24" diameter of A1
  measures "d25" diameter of A2
  measures "d35" distance of P0 L38
  measures "d39" diameter of A3
  measures "d42" angle of L36 L39 L0.start
extrude "Extrude1" add sketch "Sketch1" along normal blind 5
extrude "Extrude7" add sketch "Sketch1" along normal blind 25 contours L0 L2 L14 L30 | L0 L2 L14 L15 L22 | L0 L14 L30 | L0 L1 A0 L12 L13 L14 L15 L20 L21 L22 L23 L29 L30 L31 L32 | L2 L12 L15 L20 L23 L29 L30 A1 | L2 L13 L14 L21 L22 L31 L32 A1 | L15 L22 L30 | L14 L22 L30 | L0 L14 L22 L30 L31 | L0 L30 L31 | L2 A1 | L2 A1 | L14 L22 L31 | L15 L22 L23 L30 | L15 L23 L30 | L0 L1 A0 L13 L14 L21 L22 L31 L32 | L14 L21 L31 | L14 L21 L22 L31 | L15 L23 L29 L30 | L15 L23 L29 | L1 L2 L12 L13 L32 | L1 L2 L13 L20 | L13 L20 L32 | L12 L20 L32 | L13 L14 L21 L31 | L13 L21 L31 | L12 L15 L23 L29 | L12 L23 L29 | L12 L20 L29 L32 | L12 L20 L29 | L1 L13 L20 L21 L32 | L1 L13 L20 | L13 L21 L32 | L13 L21 L31 L32 | L12 L20 L23 L29 | L1 L20 L21
extrude "Extrude2" cut sketch "Sketch1" against normal blind 2.2 from surface at 25 contours L0 L2 L14 L30 | L0 L2 L14 L15 L22 | L0 L14 L30 | L2 L12 L15 L20 L23 L29 L30 A1 | L2 L13 L14 L21 L22 L31 L32 A1 | L15 L22 L30 | L14 L22 L30 | L0 L14 L22 L30 L31 | L0 L30 L31 | L2 A1 | L2 A1 | L14 L22 L31 | L15 L22 L23 L30 | L15 L23 L30 | L14 L21 L31 | L14 L21 L22 L31 | L15 L23 L29 L30 | L15 L23 L29 | L1 L2 L12 L13 L32 | L1 L2 L13 L20 | L13 L20 L32 | L12 L20 L32 | L13 L14 L21 L31 | L13 L21 L31 | L12 L15 L23 L29 | L12 L23 L29 | L12 L20 L29 L32 | L12 L20 L29 | L1 L13 L20 L21 L32 | L1 L13 L20 | L13 L21 L32 | L13 L21 L31 L32 | L12 L20 L23 L29 | L1 L20 L21
extrude "Extrude3" cut sketch "Sketch1" along normal blind 22.8 contours L2 A1 | L2 A1
extrude "Extrude4" add sketch "Sketch1" along normal blind 12 contours L3 L5 A2 L36 L37 L39 | L3 L5 L6 A2 L33 L37 L38 L40 | L5 L6 A2 L34 L35 L39 L40 | L5 L34 L35 L36 L37 A3 | L5 L33 L34 L37 L38 A3 | L6 A2 L40 | L5 A3 | L5 A3 | L5 L6 L40 | L5 L34 L40
extrude "Extrude5" cut sketch "Sketch1" along normal mid plane 4 from surface at 7 contours L5 L6 A2 L34 L35 L39 L40 | L5 L34 L35 L36 L37 A3 | L5 L33 L34 L37 L38 A3 | L6 A2 L40 | L5 A3 | L5 A3 | L5 L34 L40
extrude "Extrude6" cut sketch "Sketch1" along normal blind 14 contours L5 A3 | L5 A3
fillet "Fillet1" radius 20 1 edges at (10, 6, 5)
fillet "Fillet2" radius 100 2 edges at (8, 0, 12.5) (8, 12, 12.5)
equation "d13 = ( 90 / 3 ) * 1 deg"

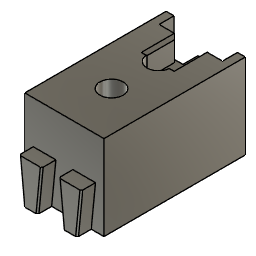
design "Connector_piece"
Autodesk Fusion 360 part; units mm, degrees
sketch "Sketch1" plane through (0, 0, 0) normal (0, 1, 0) x (1, 0, 0)
  line L0 (0, 0) -> (28, 0)
  line L1 (28, 0) -> (28, -30)
  line L2 (28, -30) -> (0, -30)
  line L3 (0, -30) -> (0, 0)
  dimension "d1" = 28
  dimension "d2" = 30
  constraint horizontal L0
  constraint vertical L1
  constraint horizontal L2
  constraint vertical L3
  constraint coincident L0.start L3.end
  measures "d1" distance of L0.start L0.end
  measures "d2" distance of L0.start L2.end
extrude "Extrude1" add sketch "Sketch1" along normal blind 50
sketch "Sketch3" plane through (0, 0, 30) normal (0, 0, 1) x (-1, 0, 0)
  line L0 (0, 0) -> (-28, 0)
  line L1 (-28, 0) -> (-28, -50)
  line L2 (-28, -50) -> (0, -50)
  line L3 (0, -50) -> (0, 0)
  line L4 (0, -16.6667) -> (-28, -16.6667)
  line L5 (0, -33.3333) -> (-28, -33.3333)
  circle A0 centre (-14, -33.3333) radius 2
  circle A1 centre (-14, -16.6667) radius 2
  circle A2 centre (-14, -16.6667) radius 4.1
  circle A3 centre (-14, -33.3333) radius 4.1
  dimension "d25" = 16.6667
  dimension "d26" = 16.6667
  dimension "d27" = 4
  dimension "d28" = 4
  dimension "d29" = 8.2
  dimension "d30" = 8.2
  constraint coincident L3 L4.start
  constraint coincident L1 L4.end
  constraint perpendicular L1 L4
  constraint coincident L3 L5.start
  constraint coincident L1 L5.end
  constraint perpendicular L1 L5
  constraint midpoint L5 A0.centre
  constraint midpoint L4 A1.centre
  constraint concentric A1 A2
  constraint concentric A0 A3
  measures "d25" distance of L0 L4
  measures "d26" distance of L2 L5
  measures "d27" diameter of A0
  measures "d28" diameter of A1
  measures "d29" diameter of A2
  measures "d30" diameter of A3
extrude "Extrude5" cut sketch "Sketch3" against normal blind 30 contours L4 A1 | L4 A1 | L5 A0 | L5 A0
sketch "Sketch2" plane through (0, 50, 0) normal (0, 1, 0) x (-1, 0, 0)
  line L0 (0, 30) -> (-28, 30)
  line L1 (-28, 30) -> (-28, 0)
  line L2 (-28, 0) -> (0, 0)
  line L3 (0, 0) -> (0, 30)
  line L4 (-28, 30) -> (-14, 30) construction
  line L5 (-14, 30) -> (-14, 0) construction
  line L6 (-14, 0) -> (-28, 0) construction
  line L7 (-28, 0) -> (-28, 30) construction
  line L8 (-21, 30) -> (-21, 0) construction
  line L9 (-21, 0) -> (-23.5, 0)
  line L10 (-21, 0) -> (-18.5, 0)
  line L11 (-21, 15) -> (-25, 15)
  line L12 (-25, 15) -> (-23.5, 0)
  line L13 (-21, 0) -> (-18.5, 0)
  line L14 (-21, 0) -> (-23.5, 0)
  line L15 (-17, 15) -> (-18.5, 0)
  line L16 (-21, 15) -> (-17, 15)
  line L17 (-11, 15) -> (-9.5, 0)
  line L18 (-7, 15) -> (-11, 15)
  line L19 (-7, 15) -> (-3, 15)
  line L20 (-3, 15) -> (-4.5, 0)
  line L21 (-7, 0) -> (-4.5, 0)
  line L22 (-7, 0) -> (-9.5, 0)
  line L23 (-21, 15.5) -> (-16.4475, 15.5)
  line L24 (-16.4475, 15.5) -> (-18.0475, -0.5)
  line L25 (-21, -0.5) -> (-18.0475, -0.5)
  line L26 (-21, -0.5) -> (-23.9525, -0.5)
  line L27 (-25.5525, 15.5) -> (-23.9525, -0.5)
  line L28 (-21, 15.5) -> (-25.5525, 15.5)
  line L29 (-7, -0.5) -> (-9.9525, -0.5)
  line L30 (-11.5525, 15.5) -> (-9.9525, -0.5)
  line L31 (-7, 15.5) -> (-11.5525, 15.5)
  line L32 (-7, 15.5) -> (-2.4475, 15.5)
  line L33 (-2.4475, 15.5) -> (-4.0475, -0.5)
  line L34 (-7, -0.5) -> (-4.0475, -0.5)
  line L35 (-25.5525, 15.5) -> (-25.5525, 30)
  line L36 (-2.4475, 15.5) -> (-2.4475, 30)
  line L37 (-16.4475, 15.5) -> (-16.4475, 30)
  line L38 (-11.5525, 15.5) -> (-11.5525, 30)
  line L39 (-28, 30) -> (-28, 22)
  line L40 (0, 30) -> (0, 22)
  line L41 (0, 22) -> (-9.2, 22)
  line L42 (-28, 22) -> (-18.8, 22)
  line L43 (-18.8, 22) -> (-18.8, 30)
  line L44 (-9.2, 22) -> (-9.2, 30)
  line L45 (-18.8, 22) -> (-9.2, 22)
  line L46 (-7, 15.2) -> (-11.221, 15.2)
  line L47 (-11.221, 15.2) -> (-9.681, -0.2)
  line L48 (-7, -0.2) -> (-9.681, -0.2)
  line L49 (-7, -0.2) -> (-4.319, -0.2)
  line L50 (-2.779, 15.2) -> (-4.319, -0.2)
  line L51 (-7, 15.2) -> (-2.779, 15.2)
  line L52 (-21, 15.2) -> (-16.779, 15.2)
  line L53 (-16.779, 15.2) -> (-18.319, -0.2)
  line L54 (-21, -0.2) -> (-18.319, -0.2)
  line L55 (-21, -0.2) -> (-23.681, -0.2)
  line L56 (-25.221, 15.2) -> (-23.681, -0.2)
  line L57 (-21, 15.2) -> (-25.221, 15.2)
  line L58 (-25.221, 15.2) -> (-25.221, 30)
  line L59 (-16.779, 15.2) -> (-16.779, 30)
  line L60 (-11.221, 15.2) -> (-11.221, 30)
  line L61 (-2.779, 15.2) -> (-2.779, 30)
  dimension "d5" = 2.5
  dimension "d6" = 2.5
  dimension "d7" = 4
  dimension "d8" = 15
  dimension "d9" = -0.5
  dimension "d16" = 8
  dimension "d17" = 8
  dimension "d18" = 9.2
  dimension "d19" = 9.2
  dimension "d20" = 8
  dimension "d37" = 0.2
  dimension "d38" = 0.2
  dimension "d39" = 180
  constraint horizontal L4
  constraint vertical L5
  constraint horizontal L6
  constraint vertical L7
  constraint midpoint L2 L5.end
  constraint coincident L0.end L1.start
  constraint midpoint L4 L8.start
  constraint midpoint L6 L8.end
  constraint perpendicular L8 L9
  constraint perpendicular L8 L10
  constraint coincident L8 L11.start
  constraint perpendicular L8 L11
  constraint symmetric L9.start L8 L10.start
  constraint symmetric L8 L9.end L10.end
  constraint symmetric L8 L10.end L9.end
  constraint symmetric L8 L11.start L16.start
  constraint symmetric L8 L11.end L15.start
  constraint symmetric L5 L8.end L21.start
  constraint symmetric L5 L9.end L20.end
  constraint symmetric L5 L11.start L18.start
  constraint symmetric L5 L11.end L19.end
  constraint symmetric L5 L10.end L17.end
  constraint symmetric L5 L15.start L17.start
  constraint vertical L35
  constraint coincident L4 L35.end
  constraint symmetric L5 L27.start L32.end
  constraint symmetric L5 L35.end L36.end
  constraint symmetric L8 L27.start L23.end
  constraint symmetric L8 L35.end L37.end
  constraint symmetric L5 L23.end L30.start
  constraint symmetric L5 L37.end L38.end
  constraint perpendicular L4 L39
  constraint coincident L0.start L3.end
  constraint perpendicular L0 L40
  constraint perpendicular L40 L41
  constraint perpendicular L35 L42
  constraint vertical L43
  constraint coincident L0 L44.end
  constraint perpendicular L0 L44
  constraint vertical L58
  constraint coincident L4 L58.end
  constraint coincident L4 L59.end
  constraint symmetric L5 L52.end L46.end
  constraint symmetric L5 L56.start L50.start
  constraint symmetric L5 L58.end L61.end
  constraint symmetric L5 L59.end L60.end
  measures "d5" distance of L8.end L9.end
  measures "d6" distance of L8.end L10.end
  measures "d7" distance of L11.start L11.end
  measures "d8" distance of L9 L11
  measures "d16" distance of L0.end L39.end
  measures "d17" distance of L0.start L40.end
  measures "d18" distance of L40.end L41.end
  measures "d19" distance of L39.end L42.end
  measures "d20" distance of L42.end L43.end
  measures "d39" angle of L58 L59
extrude "Extrude6" cut sketch "Sketch3" against normal blind 24 contours L4 A1 A2 | L4 A1 A2 | L5 A0 A3 | L5 A0 A3
chamfer "Chamfer4" distance 1.8 angle 45 2 edges at (15.8647, 34.0566, 6) (15.8647, 17.3899, 6)
extrude "Extrude4" cut sketch "Sketch2" against normal blind 16 contours L0 L44 L45 L60 | L0 L38 L45 L60 | L0 L37 L38 L45 | L0 L37 L45 L59 | L0 L43 L45 L59
extrude "Extrude3" add sketch "Sketch2" against normal blind 5 from surface at -50 contours L2 L17 L18 L19 L20 L21 L22 | L2 L9 L10 L11 L12 L13 L14 L15 L16
chamfer "Chamfer1" distance 0.5 angle 45 4 edges at (3.75, -5, 7.5) (10.25, -5, 7.5) (17.75, -5, 7.5) (24.25, -5, 7.5)
extrude "Extrude2" cut sketch "Sketch2" against normal blind 5.3 contours L0 L41 L44 L61 | L0 L44 L45 L60 | L31 L32 L41 L45 L60 L61 | L31 L32 L46 L51 L60 L61 | L2 L17 L18 L19 L20 L46 L47 L50 L51 | L2 L17 L18 L19 L20 L21 L22 | L0 L43 L45 L59 | L0 L42 L43 L58 | L23 L28 L42 L45 L58 L59 | L23 L28 L52 L57 L58 L59 | L2 L9 L10 L13 L14 L53 L54 L55 L56 | L2 L11 L12 L15 L16 L52 L53 L56 L57 | L2 L9 L10 L11 L12 L13 L14 L15 L16
chamfer "Chamfer2" distance 1 angle 45 4 edges at (18.8, 39.35, 30) (18.4227, 34, 30) (9.5773, 34, 30) (9.2, 39.35, 30)
chamfer "Chamfer3" distance 1 angle 45 2 edges at (18.8, 44.7, 25.5) (9.2, 44.7, 25.5)
chamfer "Chamfer6" distance 0.7 angle 45 2 edges at (18.0454, 34, 25.5) (9.9546, 34, 25.5)
ref_plane "WorkPlane1" through (14, 25, 15) normal (1, 0, 0) x (0, 0, -1)
equation "d25 = ( 50 / 3 ) * 1 mm"
equation "d26 = ( 50 / 3 ) * 1 mm"

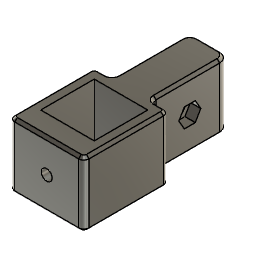
design "Pin_height_adjuster"
Autodesk Fusion 360 part; units mm, degrees
sketch "Sketch1" plane through (0, 0, 0) normal (0, 0, 1) x (1, 0, 0)
  line L0 (10, -10) -> (-10, -10)
  line L1 (-10, -10) -> (-10, 10)
  line L2 (-10, 10) -> (10, 10)
  line L3 (10, 10) -> (10, -10)
  line L4 (10, -10) -> (-10, 10) construction
  line L5 (-10, -10) -> (10, 10) construction
  line L6 (10.3, -10.3) -> (-10.3, -10.3)
  line L7 (-10.3, -10.3) -> (-10.3, 10.3)
  line L8 (-10.3, 10.3) -> (10.3, 10.3)
  line L9 (10.3, 10.3) -> (10.3, -10.3)
  line L10 (-14.3, -14.3) -> (-14.3, 14.3)
  line L11 (-14.3, 14.3) -> (14.3, 14.3)
  line L12 (14.3, 14.3) -> (14.3, -14.3)
  line L13 (14.3, -14.3) -> (-14.3, -14.3)
  line L14 (-14.3, -14.3) -> (14.3, -14.3)
  line L15 (14.3, -14.3) -> (14.3, -18.3)
  line L16 (14.3, -18.3) -> (-14.3, -18.3)
  line L17 (-14.3, -18.3) -> (-14.3, -14.3)
  dimension "d1" = 20
  dimension "d2" = 20
  dimension "d3" = -0.3
  dimension "d4" = -4.3
  dimension "d10" = 28.6
  dimension "d11" = 4
  constraint horizontal L0
  constraint perpendicular L0 L1
  constraint parallel L0 L2
  constraint parallel L1 L3
  constraint coincident L4 origin
  constraint coincident L5 origin
  constraint horizontal L14
  constraint vertical L15
  constraint horizontal L16
  constraint vertical L17
  measures "d1" distance of L1.end L2.end
  measures "d2" distance of L0.end L1.end
  measures "d10" distance of L10.start L12.end
  measures "d11" distance of L10.start L16.end
extrude "Extrude1" add sketch "Sketch1" along normal blind 25 contours L10 L11 L12 L13 L14 | L13 L14 L15 L16 L17
sketch "Sketch3" plane through (0, -10.3, 0) normal (0, 1, 0) x (-1, 0, 0)
  line L0 (-10.3, 0) -> (10.3, 0)
  line L1 (10.3, 0) -> (10.3, 25)
  line L2 (10.3, 25) -> (-10.3, 25)
  line L3 (-10.3, 25) -> (-10.3, 0)
  line L4 (-10.3, 25) -> (10.3, 25)
  line L5 (10.3, 25) -> (10.3, 0)
  line L6 (10.3, 0) -> (-10.3, 0)
  line L7 (-10.3, 0) -> (-10.3, 25)
  line L8 (-10.3, 25) -> (10.3, 0) construction
  line L9 (10.3, 25) -> (-10.3, 0) construction
  line L10 (2.1073, 8.85) -> (4.2147, 12.5)
  line L11 (4.2147, 12.5) -> (2.1073, 16.15)
  line L12 (2.1073, 16.15) -> (-2.1073, 16.15)
  line L13 (-2.1073, 16.15) -> (-4.2147, 12.5)
  line L14 (-4.2147, 12.5) -> (-2.1073, 8.85)
  line L15 (-2.1073, 8.85) -> (2.1073, 8.85)
  circle A0 centre (0, 12.5) radius 2.1
  point P0 (0, 12.5)
  dimension "d12" = 25
  dimension "d13" = 3.65
  dimension "d16" = 4.2
  constraint horizontal L4
  constraint vertical L5
  constraint horizontal L6
  constraint vertical L7
  constraint coincident L2.end L3.start
  constraint coincident L0.end L1.start
  constraint midpoint L9 P0
  constraint coincident P0 A0.centre
  measures "d12" distance of L2.end L0.start
  measures "d13" distance of P0 L15
  measures "d16" diameter of A0
extrude "Extrude4" cut sketch "Sketch3" against normal blind 8 contours A0
extrude "Extrude3" cut sketch "Sketch3" against normal blind 4 contours L10 L11 L12 L13 L14 L15 | A0
sketch "Sketch6" plane through (0, 14.3, 0) normal (0, 1, 0) x (-1, 0, 0)
  line L0 (-14.3, 0) -> (14.3, 0)
  line L1 (14.3, 0) -> (14.3, 25)
  line L2 (14.3, 25) -> (-14.3, 25)
  line L3 (-14.3, 25) -> (-14.3, 0)
  line L4 (-14.3, 25) -> (14.3, 0) construction
  line L5 (14.3, 25) -> (-14.3, 0) construction
  line L6 (7.5, 25) -> (-7.5, 25)
  line L7 (-7.5, 25) -> (-7.5, 0)
  line L8 (-7.5, 0) -> (7.5, 0)
  line L9 (7.5, 0) -> (7.5, 25)
  line L10 (7.5, 25) -> (-7.5, 0) construction
  line L11 (-7.5, 25) -> (7.5, 0) construction
  point P0 (0, 12.5)
  dimension "d35" = 15
  dimension "d36" = 25
  constraint coincident L2.end L3.start
  constraint coincident L0.end L1.start
  constraint coincident L1.end L2.start
  constraint coincident L0.start L3.end
  constraint horizontal L6
  constraint perpendicular L6 L7
  constraint parallel L6 L8
  constraint parallel L7 L9
  constraint coincident L10 P0
  constraint coincident L11 P0
  constraint midpoint L5 P0
  measures "d35" distance of L7.end L8.end
  measures "d36" distance of L6.end L7.end
extrude "Extrude10" add sketch "Sketch6" along normal blind 30 contours L0 L2 L6 L7 L8 L9
sketch "Sketch7" plane through (-7.5, 0, 0) normal (-1, 0, 0) x (0, -1, 0)
  line L0 (-14.3, 0) -> (-14.3, 25)
  line L1 (-14.3, 25) -> (-44.3, 25)
  line L2 (-44.3, 25) -> (-44.3, 0)
  line L3 (-44.3, 0) -> (-14.3, 0)
  line L4 (-14.3, 25) -> (-44.3, 0) construction
  line L5 (-44.3, 25) -> (-14.3, 0) construction
  circle A0 centre (-29.3, 12.5) radius 2.1
  line L6 (-27.1927, 8.85) -> (-25.0853, 12.5)
  line L7 (-25.0853, 12.5) -> (-27.1927, 16.15)
  line L8 (-27.1927, 16.15) -> (-31.4073, 16.15)
  line L9 (-31.4073, 16.15) -> (-33.5147, 12.5)
  line L10 (-33.5147, 12.5) -> (-31.4073, 8.85)
  line L11 (-31.4073, 8.85) -> (-27.1927, 8.85)
  line L12 (-29.3, 5.75) -> (-23.4543, 9.125)
  line L13 (-23.4543, 9.125) -> (-23.4543, 15.875)
  line L14 (-23.4543, 15.875) -> (-29.3, 19.25)
  line L15 (-29.3, 19.25) -> (-35.1457, 15.875)
  line L16 (-35.1457, 15.875) -> (-35.1457, 9.125)
  line L17 (-35.1457, 9.125) -> (-29.3, 5.75)
  line L18 (-24.4543, 15.2976) -> (-29.3, 18.0953)
  line L19 (-29.3, 18.0953) -> (-34.1457, 15.2976)
  line L20 (-34.1457, 15.2976) -> (-34.1457, 9.7024)
  line L21 (-34.1457, 9.7024) -> (-29.3, 6.9047)
  line L22 (-29.3, 6.9047) -> (-24.4543, 9.7024)
  line L23 (-24.4543, 9.7024) -> (-24.4543, 15.2976)
  point P0 (-29.3, 12.5)
  point P1 (-29.3, 12.5)
  point P2 (-29.3, 12.5)
  dimension "d43" = 4.2
  dimension "d50" = 3.65
  dimension "d54" = 6.75
  dimension "d55" = -1
  constraint coincident L0.end L1.start
  constraint coincident L2.end L3.start
  constraint coincident L1.end L2.start
  constraint coincident L0.start L3.end
  constraint midpoint L5 P2
  constraint coincident P2 P1
  measures "d43" diameter of A0
  measures "d50" distance of P2 L11
  measures "d54" distance of L12.start P2
extrude "Extrude13" cut sketch "Sketch7" along normal blind 4 from surface at -15 contours L6 L7 L8 L9 L10 L11
extrude "Extrude12" cut sketch "Sketch7" against normal blind 15 contours A0
extrude "Extrude11" add sketch "Sketch7" along normal blind 1.5 contours L12 L13 L14 L15 L16 L17
fillet "Fillet1" radius 3.5 2 edges at (-7.5, 44.3, 12.5) (7.5, 44.3, 12.5)
fillet "Fillet2" radius 2 2 edges at (-7.5, 14.3, 12.5) (7.5, 14.3, 12.5)
fillet "Fillet3" radius 2 4 edges at (-14.3, 14.3, 12.5) (-14.3, -18.3, 12.5) (14.3, -18.3, 12.5) (14.3, 14.3, 12.5)
chamfer "Chamfer1" distance 1 angle 45 32 edges at (-13.7142, -17.7142, 25) (0, -18.3, 25) (13.7142, -17.7142, 25) (14.3, -2, 25) (13.7142, 13.7142, 25) (10.9, 14.3, 25) (8.0858, 14.8858, 25) (7.5, 28.55, 25) (6.4749, 43.2749, 25) (0, 44.3, 25) (-6.4749, 43.2749, 25) (-7.5, 28.55, 25) (-8.0858, 14.8858, 25) (-10.9, 14.3, 25) (-13.7142, 13.7142, 25) (-14.3, -2, 25) (-13.7142, 13.7142, 0) (-10.9, 14.3, 0) (-8.0858, 14.8858, 0) (-7.5, 28.55, 0) (-6.4749, 43.2749, 0) (0, 44.3, 0) (6.4749, 43.2749, 0) (7.5, 28.55, 0) (8.0858, 14.8858, 0) (10.9, 14.3, 0) (13.7142, 13.7142, 0) (14.3, -2, 0) (13.7142, -17.7142, 0) (0, -18.3, 0) (-13.7142, -17.7142, 0) (-14.3, -2, 0)
equation "d35 = 28.6 mm - 4 mm - 4 mm - 0.6 mm - 5 mm"
equation "d54 = ( 13.5 / 2 ) * 1 mm"

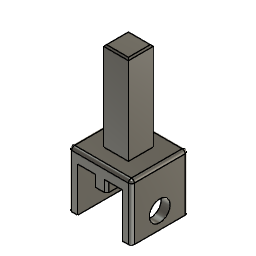
design "Slider"
Autodesk Fusion 360 part; units mm, degrees
sketch "Sketch1" plane through (0, 0, 0) normal (0, 1, 0) x (1, 0, 0)
  line L0 (0, 0) -> (6, 0)
  line L1 (6, 0) -> (6, -38)
  line L2 (6, -38) -> (0, -38)
  line L3 (0, -38) -> (0, 0)
  line L4 (0, -38) -> (42.4, -38)
  line L5 (42.4, -38) -> (42.4, -30)
  line L6 (42.4, -30) -> (0, -30)
  line L7 (0, -30) -> (0, -38)
  line L8 (42.4, -38) -> (36.4, -38)
  line L9 (36.4, -38) -> (36.4, 0)
  line L10 (36.4, 0) -> (42.4, 0)
  line L11 (42.4, 0) -> (42.4, -38)
  line L12 (16.75, -38) -> (25.65, -38)
  line L13 (25.65, -38) -> (25.65, -22.4)
  line L14 (25.65, -22.4) -> (16.75, -22.4)
  line L15 (16.75, -22.4) -> (16.75, -38)
  dimension "d1" = 6
  dimension "d2" = 38
  dimension "d3" = 8
  dimension "d5" = 6
  dimension "d6" = 38
  dimension "d8" = 15.6
  dimension "d9" = 10.75
  dimension "d29" = 10.75
  dimension "d30" = 42.4
  constraint horizontal L0
  constraint vertical L1
  constraint horizontal L2
  constraint vertical L3
  constraint coincident L0.start L3.end
  constraint horizontal L4
  constraint vertical L5
  constraint horizontal L6
  constraint vertical L7
  constraint horizontal L8
  constraint vertical L9
  constraint horizontal L10
  constraint vertical L11
  constraint horizontal L12
  constraint vertical L13
  constraint horizontal L14
  constraint vertical L15
  constraint coincident L4 L12.start
  measures "d1" distance of L0.start L0.end
  measures "d2" distance of L0.start L2.end
  measures "d3" distance of L2.end L6.end
  measures "d5" distance of L4.end L8.end
  measures "d6" distance of L4.end L10.end
  measures "d8" distance of L12.start L14.end L0.start
  measures "d9" distance of L1 L15 L0.start
  measures "d29" distance of L9 L13
  measures "d30" distance of L3 L11
extrude "Extrude1" add sketch "Sketch1" along normal blind 38.4